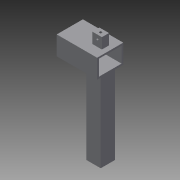
# Autodesk Inventor part: DART Actuator
Saved by Autodesk Inventor 2015 (Build 190159000, 159)
## iProperties
Created: 2015-02-14
Part Number: DART Actuator
Material: Generic
Document SubType Name: Modeling
Designer: pltwe4
Density: 1 g/cm^3
Appearance: Default
Author: pltwe4
Autodesk Inventor part; units mm, degrees
ref_plane "YZ Plane" through (0, 0, 0) normal (1, 0, 0) x (0, 1, 0)
ref_plane "XZ Plane" through (0, 0, 0) normal (0, 1, 0) x (-1, 0, 0)
ref_plane "XY Plane" through (0, 0, 0) normal (0, 0, 1) x (1, 0, 0)
sketch "Sketch1" plane through (0, 0, 0) normal (0, 1, 0) x (-1, 0, 0)
  line L0 (53.975, 34.925) -> (-53.975, 34.925)
  line L1 (-53.975, 34.925) -> (-53.975, -34.925)
  line L2 (-53.975, -34.925) -> (53.975, -34.925)
  line L3 (53.975, -34.925) -> (53.975, 34.925)
  line L4 (0, -48.895) -> (0, 48.895) projected
  line L5 (-75.565, 0) -> (75.565, 0) projected
  point P0 (0, 0)
  dimension "d0" = 69.85
  dimension "d1" = 107.95
  constraints: 8 end point, 2 parallel, 1 horizontal, 1 perpendicular, 2 other
  measures "d0" distance between parallel lines of L2 L0
  measures "d1" distance between parallel lines of L1 L3
extrude "Extrusion1" add sketch "Sketch1" along normal blind 50.8
sketch "Sketch2" plane through (0, 50.8, 0) normal (0, 1, 0) x (1, 0, 0)
  line L0 (-53.975, -34.925) -> (53.975, -34.925) projected
  line L1 (53.975, -34.925) -> (53.975, 34.925) projected
  line L2 (53.975, 34.925) -> (-53.975, 34.925) projected
  line L3 (-53.975, 34.925) -> (-53.975, -34.925) projected
  line L4 (15.875, -9.525) -> (41.275, -9.525)
  line L5 (41.275, -9.525) -> (41.275, 9.525)
  line L6 (41.275, 9.525) -> (15.875, 9.525)
  line L7 (15.875, 9.525) -> (15.875, -9.525)
  line L8 (75.565, 0) -> (-75.565, 0) projected
  circle A0 centre (28.575, 0) radius 3.175
  line L9 (28.575, -9.525) -> (28.575, 9.525) construction
  point P0 (0, 0)
  dimension "d4" = 25.4
  dimension "d5" = 19.05
  dimension "d7" = 6.35
  dimension "d29" = 12.7
  constraints: 10 end point, 3 midpoint, 2 parallel, 1 centre point, 1 horizontal, 1 perpendicular, 1 point on line, 1 other
  measures "d4" distance between parallel lines of L5 L7
  measures "d5" distance between parallel lines of L4 L6
  measures "d7" diameter of A0
  measures "d29" distance between parallel lines of L1 L5
extrude "Extrusion2" add sketch "Sketch2" along normal blind 28.575 contours L8 A0 L5 L4 L7 | L7 L6 L5 L8 A0
sketch "Sketch3" plane through (-53.975, 0, -34.925) normal (-1, 0, 0) x (0, 0, 1)
  line L0 (0, 0) -> (69.85, 0) projected
  line L1 (69.85, 0) -> (69.85, 50.8) projected
  line L2 (0, 50.8) -> (69.85, 50.8) projected
  line L3 (0, 0) -> (0, 50.8) projected
  line L4 (65.278, 4.572) -> (4.572, 4.572)
  line L5 (4.572, 4.572) -> (4.572, 46.228)
  line L6 (4.572, 46.228) -> (65.278, 46.228)
  line L7 (65.278, 46.228) -> (65.278, 4.572)
  point P0 (34.925, 0)
  dimension "d10" = 4.572
  constraints: 8 end point, 3 other
  measures "d10" distance between parallel lines of L0 L4
extrude "Extrusion3" cut sketch "Sketch3" against normal up to next contours L4 L5 L6 L7
sketch "Sketch4" plane through (0, 0, 0) normal (0, -1, 0) x (1, 0, 0)
  line L0 (-53.975, 34.925) -> (53.975, 34.925) projected
  line L1 (-53.975, -34.925) -> (-53.975, 34.925) projected
  line L2 (53.975, -34.925) -> (-53.975, -34.925) projected
  line L3 (53.975, 34.925) -> (53.975, -34.925) projected
  line L4 (9.525, -19.05) -> (47.625, -19.05)
  line L5 (47.625, -19.05) -> (47.625, 19.05)
  line L6 (47.625, 19.05) -> (9.525, 19.05)
  line L7 (9.525, 19.05) -> (9.525, -19.05)
  line L8 (-79.233, 0) -> (97.5728, 0) construction
  arc A0 (-41.275, 9.525) -> (-41.275, -9.525) centre (-41.275, 0) ccw
  arc A1 (-15.875, -9.525) -> (-15.875, 9.525) centre (-15.875, 0) ccw
  arc A2 (-41.275, -23.3807) -> (-41.275, -27.4193) centre (-41.275, -25.4) ccw
  arc A3 (-15.875, -27.4193) -> (-15.875, -23.3807) centre (-15.875, -25.4) ccw
  arc A4 (-41.275, 27.4193) -> (-41.275, 23.3807) centre (-41.275, 25.4) ccw
  arc A5 (-15.875, 23.3807) -> (-15.875, 27.4193) centre (-15.875, 25.4) ccw
  line L9 (-28.575, -34.925) -> (-28.575, 34.925) construction
  line L10 (-41.275, -25.4) -> (-41.275, 25.4) construction
  line L11 (-41.275, -27.4193) -> (-15.875, -27.4193)
  line L12 (-15.875, -23.3807) -> (-41.275, -23.3807)
  line L13 (-41.275, 23.3807) -> (-15.875, 23.3807)
  line L14 (-15.875, 27.4193) -> (-41.275, 27.4193)
  line L15 (-41.275, -9.525) -> (-15.875, -9.525)
  line L16 (-15.875, 9.525) -> (-41.275, 9.525)
  circle A6 centre (28.575, 0) radius 12.7
  line L17 (28.575, 19.05) -> (28.575, -19.05) construction
  point P0 (0, 0)
  dimension "d13" = 38.1
  dimension "d14" = 6.35
  dimension "d15" = 4.0386
  dimension "d16" = 25.4
  dimension "d17" = 25.4
  dimension "d18" = 12.7
  dimension "d19" = 19.05
  dimension "d22" = 25.4
  constraints: 26 end point, 12 point on circle, 7 centre point, 7 tangent, 5 parallel, 5 point on line, 4 equal radius, 4 midpoint, 3 horizontal, 3 perpendicular, 1 vertical, 6 other
  measures "d13" distance between parallel lines of L5 L7
  measures "d14" distance between parallel lines of L3 L5
  measures "d15" diameter of A2
  measures "d16" distance of L10.start A0.centre
  measures "d17" distance between parallel lines of L9 L1
  measures "d18" distance from line of L9 A0.centre
  measures "d19" diameter of A0
  measures "d22" diameter of A6
extrude "Extrusion4" cut sketch "Sketch4" against normal up to surface (4.572 mm away) contours L16 A1 L15 A0 | L12 A3 L11 A2 | L14 A5 L13 A4
extrude "Extrusion5" add sketch "Sketch4" along normal blind 215.9 contours L7 L6 L5 L4
sketch "Sketch5" plane through (41.275, 50.8, -9.525) normal (0, 0, -1) x (-1, 0, 0)
  line L0 (25.4, 0) -> (0, 0) projected
  line L1 (25.4, 0) -> (25.4, 28.575) projected
  line L2 (0, 28.575) -> (25.4, 28.575) projected
  line L3 (0, 0) -> (0, 28.575) projected
  circle A0 centre (12.7, 18.415) radius 3.175
  line L4 (25.4, 28.575) -> (0, 28.575) construction
  line L5 (12.7, 28.575) -> (12.7, 0) construction
  point P0 (41.275, -50.8)
  dimension "d25" = 6.35
  dimension "d26" = 10.16
  constraints: 2 end point, 2 midpoint, 1 centre point, 1 point on line
  measures "d25" diameter of A0
  measures "d26" distance from line of L2 A0.centre
extrude "Extrusion6" cut sketch "Sketch5" against normal up to surface (19.05 mm away) contours A0
body "Solid1"
